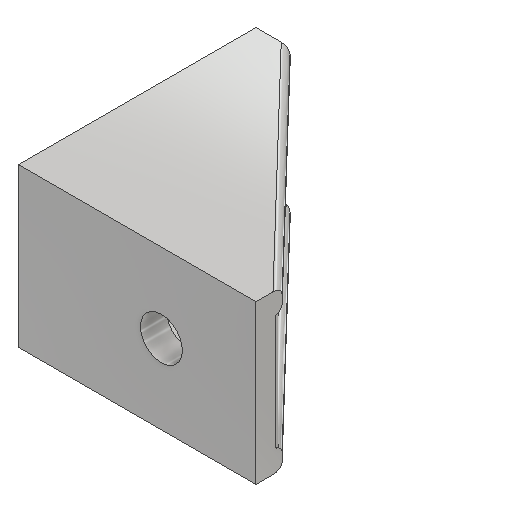
# Autodesk Inventor part: COTS_GENERIC_20x20mm_Angle_Bracket
Saved by Autodesk Inventor 2026.1 (Build 301233000, 233)
## iProperties
Created: 2017-05-11
Part Number: COTS_GENERIC_20x20mm_Angle_Bracket
Material: Stal nierdzewna 440C
Document SubType Name: Modeling
Designer: Andrzej
Density: 7.75 g/cm^3
Appearance: Aluminium - polerowane
Mass: 48.3283 g
Surface Area: 40.3171 cm^2
Volume: 6.23592 cm^3
Author: Andrzej
Autodesk Inventor part; units mm, degrees
ref_plane "YZ Plane" through (0, 0, 0) normal (1, 0, 0) x (0, 1, 0)
ref_plane "XZ Plane" through (0, 0, 0) normal (0, 1, 0) x (-1, 0, 0)
ref_plane "XY Plane" through (0, 0, 0) normal (0, 0, 1) x (1, 0, 0)
sketch "Szkic1" plane through (0, 0, 0) normal (0, 0, 1) x (1, 0, 0)
  line L0 (-7.0726, 6.5674) -> (-7.0726, -23.4326)
  line L1 (-7.0726, -23.4326) -> (22.9274, -23.4326)
  line L2 (22.9274, -23.4326) -> (22.9274, -20.1326)
  line L3 (-7.0726, 6.5674) -> (-2.7726, 6.5674)
  line L4 (-2.7726, 6.5674) -> (22.9274, -20.1326)
  point P0 (0, 0)
  dimension "d0" = 30
  dimension "d1" = 30
  dimension "d2" = 3.3
  dimension "d3" = 4.3
  constraints: 10 end point, 2 perpendicular, 1 horizontal, 1 vertical
  measures "d0" distance of L0.start L0.end
  measures "d1" distance of L0.end L1.end
  measures "d2" distance of L1.end L2.end
  measures "d3" distance of L0.start L3.end
extrude "Wyciągnięcie proste1" add sketch "Szkic1" along normal blind 20
sketch "Szkic2" plane through (22.9274, -23.4326, 0) normal (1, 0, 0) x (0, 0, -1)
  line L0 (0, 0) -> (0, 3.3) projected
  line L1 (0, 3.3) -> (-20, 3.3) projected
  line L2 (-20, 0) -> (-20, 3.3) projected
  line L3 (0, 0) -> (-20, 0) projected
  line L4 (0, 3.3) -> (0, 30) projected
  line L5 (0, 30) -> (-20, 30) projected
  line L6 (-20, 3.3) -> (-20, 30) projected
  line L7 (0, 3.3) -> (-20, 3.3) projected
  line L8 (0, 3.3) -> (-20, 3.3) projected
  line L9 (0, 30) -> (-20, 30) projected
  line L10 (-4, 3.3) -> (-16, 3.3)
  line L11 (-16, 3.3) -> (-16, 30)
  line L12 (-16, 30) -> (-4, 30)
  line L13 (-4, 30) -> (-4, 3.3)
  point P0 (0, 23.4326)
  dimension "d6" = 12
  dimension "d7" = 4
  dimension "d8" = 4
  constraints: 8 end point, 2 parallel, 2 point on line, 1 horizontal, 1 perpendicular
  measures "d6" distance of L11.end L12.end
  measures "d7" distance between parallel lines of L6 L11
  measures "d8" distance between parallel lines of L4 L13
extrude "Wyciągnięcie proste2" cut sketch "Szkic2" against normal blind 25.7 contours L1 L11 L5 L13
chamfer "Faza1" distance 1.3 distance2 18.5 1 edges at (10.0774, -6.7826, 16) measured on face at (14.3607, -11.2326, 17.3333)
chamfer "Faza2" distance 1.3 distance2 18.5 1 edges at (10.0774, -6.7826, 4) measured on face at (5.7941, -2.3326, 2.6667)
fillet "Zaokrąglenie1" radius 0.8 4 edges at (10.0774, -6.7826, 17.3) (10.0774, -6.7826, 2.7) (10.0774, -6.7826, 20) (10.0774, -6.7826, 0)
fillet "Zaokrąglenie2" radius 0.8 2 edges at (22.9274, -20.1326, 10) (-2.7726, 6.5674, 10)
sketch "Szkic3" plane through (-7.0726, -23.4326, 0) normal (0, -1, 0) x (1, 0, 0)
  line L0 (0, 0) -> (30, 0) projected
  line L1 (30, 0) -> (30, 20) projected
  line L2 (0, 20) -> (30, 20) projected
  line L3 (0, 0) -> (0, 20) projected
  point P0 (7.0726, 0)
  point P1 (18.05, 10)
  dimension "d19" = 11.95
  measures "d19" distance from line of L1 point (18.05, 10)
hole "Otwór1" at (10.9774, -23.4326, 10) direction (0, 1, 0) diameter 5.3 end through all
sketch "Szkic4" plane through (-7.0726, -23.4326, 0) normal (-1, 0, 0) x (0, 0, 1)
  line L0 (0, 30) -> (0, 0) projected
  line L1 (0, 0) -> (20, 0) projected
  line L2 (20, 30) -> (20, 0) projected
  line L3 (0, 30) -> (20, 30) projected
  point P0 (0, 23.4326)
  point P1 (10, 18.05)
  dimension "d27" = 11.95
  measures "d27" distance from line of L3 point (10, 18.05)
hole "Otwór2" at (-7.0726, -5.3826, 10) direction (1, 0, 0) diameter 5.3 end through all
